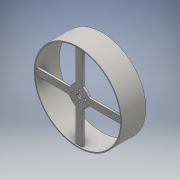
# Autodesk Inventor part: Motor mount (plain)
Saved by Autodesk Inventor 2016 (Build 200138000, 138)
## iProperties
Created: 2016-03-10
Part Number: Motor mount (plain)
Material: Generic
Document SubType Name: Modeling
Designer: s_sud
Density: 1 g/cm^3
Appearance: Default
Author: s_sud
Autodesk Inventor part; units mm, degrees
ref_plane "YZ Plane" through (0, 0, 0) normal (1, 0, 0) x (0, 1, 0)
ref_plane "XZ Plane" through (0, 0, 0) normal (0, 1, 0) x (-1, 0, 0)
ref_plane "XY Plane" through (0, 0, 0) normal (0, 0, 1) x (1, 0, 0)
sketch "Sketch1" plane through (0, 0, 0) normal (0, 1, 0) x (-1, 0, 0)
  circle A0 centre (0, 0) radius 65
  circle A1 centre (0, 0) radius 66.5
  dimension "d0" = 130
  dimension "d1" = 133
  constraints: 2 centre point, 2 coincident
  measures "d0" diameter of A0
  measures "d1" diameter of A1
extrude "Extrusion1" add sketch "Sketch1" along normal blind 35
sketch "Sketch2" plane through (0, 0, 0) normal (0, -1, 0) x (1, 0, 0)
  line L0 (5, 65.5) -> (-5, 65.5)
  line L1 (-5, -65.5) -> (5, -65.5)
  line L2 (65.5, 5) -> (65.5, -5)
  line L3 (-65.5, -5) -> (-65.5, 5)
  circle A0 centre (0, 0) radius 65 projected
  line L4 (64.8114, -4.9474) -> (65.5, -5) construction
  line L5 (65.5, 5) -> (64.8114, 4.9474) construction
  line L6 (-65.5, 5) -> (-64.8114, 4.9474) construction
  line L7 (0, 0) -> (5, -0.3817) construction
  line L8 (0, 0) -> (-5, -0.3817) construction
  line L9 (-64.8114, -4.9474) -> (-65.5, -5) construction
  line L10 (5, 65.5) -> (4.9474, 64.8114) construction
  line L11 (-5, 65.5) -> (-4.9474, 64.8114) construction
  arc A1 (14.1421, 5) -> (5, 14.1421) centre (0, 0) ccw
  arc A2 (-5, 14.1421) -> (-14.1421, 5) centre (0, 0) ccw
  line L12 (0, 0) -> (-0.3817, -5) construction
  line L13 (-4.9474, -64.8114) -> (-5, -65.5) construction
  line L14 (4.9474, -64.8114) -> (5, -65.5) construction
  arc A3 (-14.1421, -5) -> (-5, -14.1421) centre (0, 0) ccw
  arc A4 (5, -14.1421) -> (14.1421, -5) centre (0, 0) ccw
  line L15 (65.5, -5) -> (14.1421, -5)
  line L16 (5, -65.5) -> (5, -14.1421)
  line L17 (5, -0.3817) -> (5, 0.3817)
  line L18 (5, 14.1421) -> (5, 65.5)
  line L19 (-65.5, 5) -> (-14.1421, 5)
  line L20 (14.1421, 5) -> (65.5, 5)
  line L21 (-5, 65.5) -> (-5, 14.1421)
  line L22 (-5, 0.3817) -> (-5, -0.3817)
  line L23 (-5, -5) -> (-5, -65.5)
  line L24 (0.3817, -5) -> (-0.3817, -5)
  line L25 (-14.1421, -5) -> (-65.5, -5)
  dimension "d4" = 10
  dimension "d5" = 131
  dimension "d6" = 131
  dimension "d7" = 10
  constraints: 52 end point, 17 parallel, 8 point on circle, 5 perpendicular, 4 centre point, 4 point on line, 3 horizontal, 1 coincident, 9 other
  measures "d4" distance of L1.end L1.start
  measures "d5" distance of L0.end L1.start
  measures "d6" distance of L2.end L3.start
  measures "d7" distance of L3.start L3.end
extrude "Extrusion2" add sketch "Sketch2" against normal blind 3 contours L18 A0 L21 L0 | L18 A1 L20 A0 L15 A4 L16 L23 A3 L25 L19 A2 L21 | L20 L2 L15 A0 | A0 L25 L3 L19 | A0 L16 L1 L23
sketch "Sketch3" plane through (0, 0, 0) normal (0, -1, 0) x (1, 0, 0)
  circle A0 centre (0, -8) radius 1.5
  circle A1 centre (0, 8) radius 1.5
  circle A2 centre (9.5, 0) radius 1.5
  circle A3 centre (-9.5, 0) radius 1.5
  circle A4 centre (0, 0) radius 3.5464
  dimension "d11" = 3
  dimension "d12" = 8
  dimension "d13" = 3
  dimension "d14" = 9.5
  constraints: 5 centre point, 1 coincident
  measures "d11" diameter of A0
  measures "d12" distance of point (0, 0) A0.centre
  measures "d13" diameter of A2
  measures "d14" distance of point (0, 0) A2.centre
extrude "Extrusion3" cut sketch "Sketch3" against normal blind 3
sketch "Sketch4" plane through (0, 0, 0) normal (0, -1, 0) x (1, 0, 0)
  circle A0 centre (0, 0) radius 66.5 projected
  circle A1 centre (0, 0) radius 65
  dimension "d17" = 130
  constraints: 1 centre point, 1 coincident
  measures "d17" diameter of A1
extrude "Extrusion4" add sketch "Sketch4" along normal blind 2
body "Solid1"
